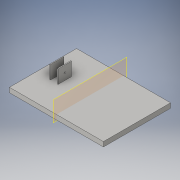
# Autodesk Inventor part: ExampleOfUsingSnowBlowerMotor
Saved by Autodesk Inventor 2016 SP1 (Build 200210100, 210)
## iProperties
Created: 2016-01-25
Part Number: ExampleOfUsingSnowBlowerMotor
Material: Generic
Document SubType Name: Modeling
Designer: steele
Density: 1 g/cm^3
Appearance: Default
Author: steele
Autodesk Inventor part; units mm, degrees
ref_plane "XZ Plane" through (0, 0, 0) normal (0, 1, 0) x (-1, 0, 0)
ref_plane "XY Plane" through (0, 0, 0) normal (0, 0, 1) x (1, 0, 0)
sketch "Sketch1" plane through (0, 0, 0) normal (0, 1, 0) x (-1, 0, 0)
  line L0 (-177.8, 127) -> (-177.8, -127)
  line L1 (-177.8, -127) -> (177.8, -127)
  line L2 (177.8, -127) -> (177.8, 127)
  line L3 (177.8, 127) -> (-177.8, 127)
  line L4 (-177.8, 127) -> (177.8, -127) construction
  line L5 (-177.8, -127) -> (177.8, 127) construction
  point P0 (0, 0)
  dimension "d0" = 355.6
  dimension "d1" = 254
  constraints: 12 end point, 2 midpoint, 2 parallel, 1 perpendicular, 1 vertical
  measures "d0" distance of L0.end L1.end
  measures "d1" distance of L0.start L0.end
extrude "Extrusion1" add sketch "Sketch1" against normal blind 17.78
sketch "Sketch3" plane through (0, 0, 0) normal (0, 1, 0) x (1, 0, 0)
  line L0 (-177.8, -127) -> (-177.8, 127) construction
  line L1 (-177.8, 0) -> (177.8, 0) construction
  line L2 (177.8, 127) -> (177.8, -127) construction
  line L3 (-127, -25.4) -> (-123.825, -25.4)
  line L4 (-123.825, -25.4) -> (-123.825, 25.4)
  line L5 (-123.825, 25.4) -> (-127, 25.4)
  line L6 (-127, 25.4) -> (-127, -25.4)
  line L7 (-127, -25.4) -> (-123.825, 25.4) construction
  line L8 (-123.825, -25.4) -> (-127, 25.4) construction
  line L9 (-98.425, -25.4) -> (-95.25, -25.4)
  line L10 (-95.25, -25.4) -> (-95.25, 25.4)
  line L11 (-95.25, 25.4) -> (-98.425, 25.4)
  line L12 (-98.425, 25.4) -> (-98.425, -25.4)
  line L13 (-98.425, -25.4) -> (-95.25, 25.4) construction
  line L14 (-95.25, -25.4) -> (-98.425, 25.4) construction
  line L15 (-177.8, 127) -> (177.8, 127) construction
  line L16 (0, 127) -> (0, -127) construction
  line L17 (177.8, -127) -> (-177.8, -127) construction
  point P0 (0, 0)
  point P1 (-125.4125, 0)
  point P2 (-96.8375, 0)
  dimension "d4" = 50.8
  dimension "d5" = 3.175
  dimension "d6" = 50.8
  dimension "d7" = 25.4
  constraints: 28 end point, 8 midpoint, 4 parallel, 2 equal length, 2 perpendicular, 2 point on line
  measures "d4" distance between parallel lines of L0 L6
  measures "d5" distance of L3.start L3.end
  measures "d6" distance of L5.end L3.start
  measures "d7" distance between parallel lines of L4 L12
extrude "Extrusion2" add sketch "Sketch3" along normal blind 50.8
sketch "Sketch4" plane through (-127, 0, -25.4) normal (-1, 0, 0) x (0, 0, 1)
  line L0 (25.4, 0) -> (25.4, 50.8) construction
  line L1 (50.8, 50.8) -> (0, 50.8) construction
  circle A0 centre (25.4, 25.4) radius 3.175
  dimension "d10" = 6.35
  dimension "d11" = 25.4
  constraints: 2 end point, 2 midpoint, 1 centre point
  measures "d10" diameter of A0
  measures "d11" distance from line of A0.centre L1
extrude "Extrusion3" cut sketch "Sketch4" against normal through all
equation "\"d0\" = plateWidth"
equation "\"d1\" = plateLength"
equation "\"d2\" = plateThickness"
equation "\"d4\" = bracketDistanceFromEdge"
equation "\"d5\" = bracketWidth"
equation "\"d6\" = bracketLength"
equation "\"d8\" = bracketHeight"
equation "\"d10\" = axelDiam"
equation "\"d11\" = axelHoleDistanceFromTopOfBracket"
equation "\"d12\" = bracketHeight"
equation "\"plateWidth\" = 355.6"
equation "\"plateLength\" = 254"
equation "\"plateThickness\" = 17.78"
equation "\"bracketDistanceFromEdge\" = 50.8"
equation "\"bracketWidth\" = 3.175"
equation "\"bracketHeight\" = 50.8"
equation "\"bracketLength\" = 50.8"
equation "\"axelDiam\" = 6.35"
equation "\"axelHoleDistanceFromTopOfBracket\" = 25.4"
body "Solid1"
